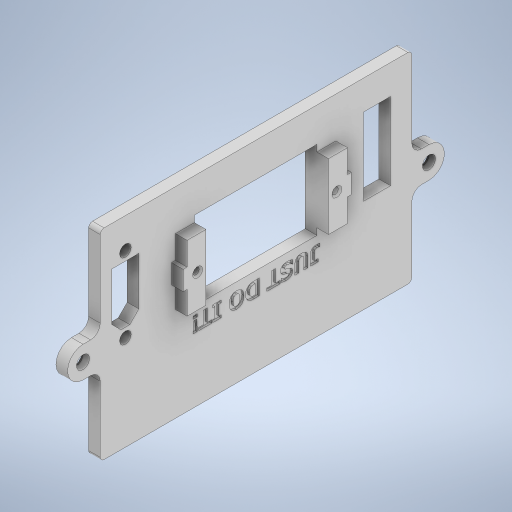
# Autodesk Inventor part: pokrywa_tyl
Saved by Autodesk Inventor 2023.4 (Build 274418000, 418)
## iProperties
Created: 2024-07-28
Part Number: pokrywa_tyl
Material: Ogólny
Document SubType Name: Modeling
Designer: kamil
Density: 1 g/cm^3
Appearance: Domyślna
Author: kamil
Autodesk Inventor part; units mm, degrees
ref_plane "YZ Plane" through (0, 0, 0) normal (1, 0, 0) x (0, 1, 0)
ref_plane "XZ Plane" through (0, 0, 0) normal (0, 1, 0) x (-1, 0, 0)
ref_plane "XY Plane" through (0, 0, 0) normal (0, 0, 1) x (1, 0, 0)
sketch "Szkic1" plane through (0, 0, 0) normal (1, 0, 0) x (0, 1, 0)
  line L0 (-29.4319, -23.6453) -> (19.8681, -23.6453)
  line L1 (19.8681, -23.6453) -> (19.8681, 56.9547)
  line L2 (19.8681, 56.9547) -> (-29.4319, 56.9547)
  line L3 (-29.4319, 56.9547) -> (-29.4319, -23.6453)
  point P0 (0, 0)
  dimension "d0" = 80.6
  dimension "d1" = 49.3
  constraints: 8 end point, 2 parallel, 1 horizontal, 1 perpendicular
  measures "d0" distance of L0.end L1.end
  measures "d1" distance between parallel lines of L3 L1
extrude "Wyciągnięcie proste1" add sketch "Szkic1" along normal blind 3
sketch "Sketch6" plane through (0, 0, 0) normal (-1, 0, 0) x (0, 0, 1)
  arc A0 (-28.0945, -0.5319) -> (-28.0945, -9.0319) centre (-28.0945, -4.7819) ccw
  line L0 (-26.3445, -9.0319) -> (-28.0945, -9.0319)
  line L1 (-26.3445, -0.5319) -> (-28.0945, -0.5319)
  line L2 (59.654, -6.3319) -> (61.404, -6.3319)
  arc A1 (61.404, -6.3319) -> (61.404, 2.1681) centre (61.404, -2.0819) ccw
  line L3 (59.654, 2.1681) -> (61.404, 2.1681)
  line L4 (-23.6453, 19.8681) -> (56.9547, 19.8681)
  line L5 (-23.6453, -29.4319) -> (-23.6453, 19.8681)
  line L6 (56.9547, -29.4319) -> (-23.6453, -29.4319)
  line L7 (56.9547, 19.8681) -> (56.9547, -29.4319)
  line L8 (-26.3445, -8.7819) -> (-28.0945, -8.7819)
  arc A2 (-28.0945, -0.7819) -> (-28.0945, -8.7819) centre (-28.0945, -4.7819) ccw
  line L9 (-28.0945, -0.7819) -> (-26.3445, -0.7819)
  line L10 (-26.3445, -0.7819) -> (-23.6453, -0.7819)
  line L11 (-23.6453, -29.4319) -> (-23.6453, 19.8681)
  line L12 (-26.3445, -8.7819) -> (-23.6453, -8.7819)
  line L13 (-23.6453, 19.8681) -> (56.9547, 19.8681)
  line L14 (16.6547, 19.8681) -> (16.6547, -29.4319)
  line L15 (56.9547, -29.4319) -> (-23.6453, -29.4319)
  line L16 (59.654, -8.7819) -> (61.404, -8.7819)
  arc A3 (61.404, -8.7819) -> (61.404, -0.7819) centre (61.404, -4.7819) ccw
  line L17 (61.404, -0.7819) -> (59.654, -0.7819)
  line L18 (59.654, -0.7819) -> (56.9547, -0.7819)
  line L19 (59.654, -8.7819) -> (56.9547, -8.7819)
  point P0 (0, 0)
extrude "Extrusion4" add sketch "Sketch6" against normal blind 3 contours L5 L12 L8 A2 L9 L10 | L18 L17 A3 L16 L19 L7
fillet "Fillet2" radius 2.5 4 edges at (1.5, -0.7819, -23.6453) (1.5, -8.7819, -23.6453) (1.5, -0.7819, 56.9547) (1.5, -8.7819, 56.9547)
sketch "Sketch8" plane through (0, 0, 0) normal (-1, 0, 0) x (0, 0, 1)
  line L0 (32.3929, 13.5523) -> (1.0929, 13.5523) projected
  line L1 (1.0929, 13.5523) -> (1.0929, -6.4477) projected
  line L2 (1.0929, -6.4477) -> (32.3929, -6.4477) projected
  line L3 (32.3929, -6.4477) -> (32.3929, 13.5523) projected
  line L4 (0.8929, -6.6477) -> (0.8929, 13.7523)
  line L5 (0.8929, 13.7523) -> (32.5929, 13.7523)
  line L6 (32.5929, 13.7523) -> (32.5929, -6.6477)
  line L7 (32.5929, -6.6477) -> (0.8929, -6.6477)
  point P0 (0, 0)
  dimension "d38" = 0.2
  constraints: 8 end point, 3 other
  measures "d38" distance between parallel lines of L1 L4
extrude "Extrusion5" cut sketch "Sketch8" against normal blind 3 contours L3 L2 L1 L0 | L4 L5 L6 L7
sketch "Sketch9" plane through (3, 0, 0) normal (1, 0, 0) x (0, 0, -1)
  line L0 (-32.5929, 13.7523) -> (-0.8929, 13.7523) projected
  line L1 (-0.8929, 13.7523) -> (-0.8929, -6.6477) projected
  line L2 (-0.8929, -6.6477) -> (-32.5929, -6.6477) projected
  line L3 (-32.5929, -6.6477) -> (-32.5929, 13.7523) projected
  line L4 (-56.9547, -29.4319) -> (23.6453, -29.4319) projected
  line L5 (23.6453, -29.4319) -> (23.6453, -11.2819) projected
  arc A0 (26.1453, -8.7819) -> (23.6453, -11.2819) centre (26.1453, -11.2819) ccw projected
  line L6 (26.1453, -8.7819) -> (28.0945, -8.7819) projected
  arc A1 (28.0945, -8.7819) -> (28.0945, -0.7819) centre (28.0945, -4.7819) ccw projected
  line L7 (28.0945, -0.7819) -> (26.1453, -0.7819) projected
  arc A2 (23.6453, 1.7181) -> (26.1453, -0.7819) centre (26.1453, 1.7181) ccw projected
  line L8 (23.6453, 1.7181) -> (23.6453, 19.8681) projected
  line L9 (23.6453, 19.8681) -> (-56.9547, 19.8681) projected
  line L10 (-56.9547, 19.8681) -> (-56.9547, 1.7181) projected
  line L11 (-37.4929, 12.0523) -> (-37.4929, 6.0523) projected
  line L12 (-37.4929, 6.0523) -> (-38.4929, 6.0523) projected
  line L13 (-38.4929, 6.0523) -> (-38.4929, 1.0523) projected
  line L14 (-38.4929, 1.0523) -> (-37.4929, 1.0523) projected
  line L15 (-37.4929, 1.0523) -> (-37.4929, -4.9477) projected
  line L16 (-37.4929, -4.9477) -> (4.0071, -4.9477) projected
  line L17 (4.0071, -4.9477) -> (4.0071, 1.0523) projected
  line L18 (4.0071, 1.0523) -> (5.0071, 1.0523) projected
  line L19 (5.0071, 1.0523) -> (5.0071, 6.0523) projected
  line L20 (5.0071, 6.0523) -> (4.0071, 6.0523) projected
  line L21 (4.0071, 6.0523) -> (4.0071, 12.0523) projected
  line L22 (4.0071, 12.0523) -> (-37.4929, 12.0523) projected
  circle A3 centre (1.2571, 3.5523) radius 1.2 projected
  circle A4 centre (-34.7429, 3.5523) radius 1.2 projected
  line L23 (-59.4547, -0.7819) -> (-61.404, -0.7819) projected
  arc A5 (-61.404, -0.7819) -> (-61.404, -8.7819) centre (-61.404, -4.7819) ccw projected
  line L24 (-61.404, -8.7819) -> (-59.4547, -8.7819) projected
  line L25 (-56.9547, -11.2819) -> (-56.9547, -29.4319) projected
  arc A6 (-59.4547, -0.7819) -> (-56.9547, 1.7181) centre (-59.4547, 1.7181) ccw projected
  arc A7 (-56.9547, -11.2819) -> (-59.4547, -8.7819) centre (-59.4547, -11.2819) ccw projected
  point P0 (0, 0)
  point P1 (-0.8929, 12.0523)
  point P2 (-0.8929, -4.9477)
  point P3 (-32.5929, -4.9477)
  point P4 (-32.5929, 12.0523)
ref_plane "Work Plane2" through (6, -4.9477, 32.3929) normal (-1, 0, 0) x (0, 0, 1)
extrude "Extrusion6" add sketch "Sketch9" along normal up to surface (3 mm away) contours L3 L16 L15 L14 L13 L12 L11 L22 | L22 L21 L20 L19 L18 L17 L16 L1 | A3 | A4
sketch "Sketch10" plane through (6, -4.9477, 32.5929) normal (1, 0, 0) x (0, 0, -1)
  circle A0 centre (33.85, 8.5) radius 1.2 projected
  circle A1 centre (-2.15, 8.5) radius 1.2 projected
  point P0 (32.5929, 4.9477)
hole "Hole4" at (6, 3.5523, -1.2571) at (6, 3.5523, 34.7429) direction (-1, 0, 0) diameter 1.7 depth 5 tip angle 118 countersink diameter 2.6 countersink angle 90
sketch "Sketch12" plane through (0, 0, 0) normal (-1, 0, 0) x (0, 0, 1)
  arc A0 (-28.0945, -0.7819) -> (-28.0945, -8.7819) centre (-28.0945, -4.7819) ccw projected
  arc A1 (61.404, -8.7819) -> (61.404, -0.7819) centre (61.404, -4.7819) ccw projected
  point P0 (0, 0)
hole "Hole5" at (0, -4.7819, -28.0945) at (0, -4.7819, 61.404) direction (1, 0, 0) diameter 3.4 depth 10 countersink diameter 6 countersink angle 90
sketch "Sketch13" plane through (0, -29.4319, -23.6453) normal (0, -1, 0) x (1, 0, 0)
  line L0 (0, 80.6) -> (0, 0) projected
  line L1 (0, 0) -> (3, 0) projected
  line L2 (3, 80.6) -> (3, 0) projected
  line L3 (0, 80.6) -> (3, 80.6) projected
  point P0 (0, 23.6453)
extrude "Extrusion8" add sketch "Sketch13" along normal blind 2.7
sketch "Sketch14" plane through (3, 0, 0) normal (1, 0, 0) x (0, 0, -1)
  line L0 (-56.9547, -11.2819) -> (-56.9547, -32.1319) projected
  line L1 (23.6453, -32.1319) -> (-56.9547, -32.1319) projected
  line L2 (23.6453, -11.2819) -> (23.6453, -32.1319) projected
  line L3 (-56.9547, -32.1319) -> (23.6453, -32.1319)
  line L4 (23.6453, -32.1319) -> (23.6453, -29.3319)
  line L5 (23.6453, -29.3319) -> (-56.9547, -29.3319)
  line L6 (-56.9547, -29.3319) -> (-56.9547, -32.1319)
  point P0 (0, 0)
  dimension "d70" = 2.8
  constraints: 8 end point, 2 parallel, 1 horizontal, 1 perpendicular, 1 point on line
  measures "d70" distance between parallel lines of L1 L5
extrude "Extrusion9" cut sketch "Sketch14" against normal through all
sketch "Sketch15" plane through (0, 19.8681, 56.9547) normal (0, 1, 0) x (1, 0, 0)
  line L0 (0, 80.6) -> (0, 0) projected
  line L1 (0, 0) -> (3, 0) projected
  line L2 (3, 80.6) -> (3, 0) projected
  line L3 (0, 80.6) -> (3, 80.6) projected
  point P0 (0, 56.9547)
extrude "Extrusion10" add sketch "Sketch15" along normal blind 2.7
fillet "Fillet7" radius 1 4 edges at (1.5, 22.5681, 56.9547) (1.5, 22.5681, -23.6453) (1.5, -29.3319, -23.6453) (1.5, -29.3319, 56.9547)
sketch "Sketch16" plane through (0, 0, 0) normal (-1, 0, 0) x (0, 0, 1)
  line L0 (-11.1453, -5.0319) -> (-18.1453, -5.0319)
  line L1 (-18.1453, -5.0319) -> (-18.1453, 14.9681)
  line L2 (-18.1453, 14.9681) -> (-11.1453, 14.9681)
  line L3 (-11.1453, 14.9681) -> (-11.1453, -5.0319)
  line L4 (50.4547, 14.7181) -> (50.4547, -4.7819) construction
  circle A0 centre (50.4547, 14.7181) radius 1.5
  circle A1 centre (50.4547, -4.7819) radius 1.5
  line L5 (53.9547, 12.3681) -> (53.9547, -2.4319)
  line L6 (53.9547, -2.4319) -> (46.9547, -2.4319)
  line L7 (46.9547, -2.4319) -> (46.9547, 12.3681)
  line L8 (46.9547, 12.3681) -> (53.9547, 12.3681)
  line L9 (50.4547, 8.5681) -> (50.4547, 1.3681)
  circle A2 centre (50.4547, 8.5681) radius 2.25
  circle A3 centre (50.4547, 1.3681) radius 2.25
  line L10 (46.9547, -0.0816) -> (49.305, -2.4319)
  line L11 (53.9547, -0.0816) -> (51.6045, -2.4319)
  circle A4 centre (50.4547, 1.3681) radius 3.5
  line L12 (56.9547, -11.2819) -> (56.9547, -28.3319) projected
  line L13 (-22.6453, -29.3319) -> (55.9547, -29.3319) projected
  line L14 (-23.6453, -11.2819) -> (-23.6453, -28.3319) projected
  circle A5 centre (61.404, -4.7819) radius 1.7 projected
  point P0 (0, 0)
  point P1 (50.4547, 4.9681)
  point P2 (53.9547, 4.9681)
  point P3 (50.4547, 4.9681)
  point P4 (50.4547, 12.3681)
  point P5 (13.6547, 4.9681)
  point P6 (-11.1453, 4.9681)
  point P7 (-14.6453, -5.0319)
  point P8 (16.6547, -29.3319)
  dimension "d76" = 7
  dimension "d77" = 20
  dimension "d78" = 19.5
  dimension "d79" = 3
  dimension "d80" = 3
  dimension "d81" = 14.8
  dimension "d82" = 7
  dimension "d83" = 7.2
  dimension "d84" = 4.5
  dimension "d85" = 4.5
  dimension "d86" = 45
  dimension "d87" = 45
  dimension "d98" = 3
  dimension "d99" = 45
  dimension "d101" = 5.5
  constraints: 24 end point, 7 midpoint, 5 centre point, 5 coincident, 5 horizontal alignment, 5 parallel, 4 point on line, 3 perpendicular, 3 tangent, 3 vertical alignment, 1 horizontal
  measures "d76" distance of L1.end L2.end
  measures "d77" distance of L0.end L1.end
  measures "d78" distance of L4.start L4.end
  measures "d79" diameter of A0
  measures "d80" diameter of A1
  measures "d81" distance of L6.end L7.end
  measures "d82" distance of L5.end L6.end
  measures "d83" distance of L9.start L9.end
  measures "d84" diameter of A2
  measures "d85" diameter of A3
  measures "d86" angle of L5 L11
  measures "d87" angle of L7 L10
  measures "d98" distance between parallel lines of L5 L12
  measures "d99" angle of L6 L11
  measures "d101" distance between parallel lines of L14 L1
extrude "Extrusion11" cut sketch "Sketch16" against normal through all contours L0 L1 L2 L3 | A0 | A1 | L5 A4 L7 L8 | A4 | L5 L11 A4 | L11 L6 L10 A4 | A4 L10 L7 | A2 | A3
sketch "Sketch17" plane through (3, 0, 0) normal (1, 0, 0) x (0, 0, -1)
  line L0 (5.0407, -18.26) -> (-38.5266, -18.26) construction
  line L1 (-38.5266, -18.26) -> (-38.5266, -3.1594) construction
  line L2 (-38.5266, -3.1594) -> (5.0407, -3.1594) construction
  line L3 (5.0407, -3.1594) -> (5.0407, -18.26) construction
  line L4 (-0.8929, -6.6477) -> (-32.5929, -6.6477) projected
  spline S0 degree 2 poles (-2.529, -9.8831) (-2.529, -9.6238) (-2.3507, -9.1635) (-2.1724, -9.0014) knots 0 0 0 1 2 2 2
  spline S1 degree 2 poles (-2.1724, -9.0014) (-1.9715, -8.8199) (-1.4237, -8.6481) (-1.0671, -8.6481) knots 0 0 0 1 2 2 2
  spline S2 degree 2 poles (-1.0671, -8.6481) (-0.8013, -8.6481) (-0.3345, -8.687) (-0.1562, -8.7259) knots 0 0 0 1 2 2 2
  line L5 (-0.1562, -8.7259) -> (-0.1562, -9.5362)
  line L6 (-0.1562, -9.5362) -> (-0.247, -9.5362)
  spline S3 degree 2 poles (-0.247, -9.5362) (-0.3669, -9.4876) (-0.6295, -9.4033) (-0.8369, -9.4033) knots 0 0 0 1 2 2 2
  spline S4 degree 2 poles (-0.8369, -9.4033) (-1.1028, -9.4033) (-1.3912, -9.5525) (-1.4496, -9.6886) knots 0 0 0 1 2 2 2
  spline S5 degree 2 poles (-1.4496, -9.6886) (-1.5112, -9.8215) (-1.5241, -10.1651) (-1.5241, -10.379) knots 0 0 0 1 2 2 2
  line L7 (-1.5241, -10.379) -> (-1.5241, -11.9836)
  line L8 (-1.5241, -11.9836) -> (-0.61, -11.9836)
  line L9 (-0.61, -11.9836) -> (-0.61, -12.7097)
  line L10 (-0.61, -12.7097) -> (-2.529, -12.7097)
  line L11 (-2.529, -12.7097) -> (-2.529, -9.8831)
  spline S6 degree 2 poles (-4.9245, -8.6254) (-4.1173, -8.6254) (-3.2486, -9.4033) (-3.2486, -10.1554) knots 0 0 0 1 2 2 2
  line L12 (-3.2486, -10.1554) -> (-3.2486, -12.7097)
  line L13 (-3.2486, -12.7097) -> (-4.2535, -12.7097)
  line L14 (-4.2535, -12.7097) -> (-4.2535, -10.2137)
  spline S7 degree 2 poles (-4.2535, -10.2137) (-4.2535, -9.7956) (-4.5679, -9.3871) (-4.9245, -9.3871) knots 0 0 0 1 2 2 2
  spline S8 degree 2 poles (-4.9245, -9.3871) (-5.2713, -9.3871) (-5.5955, -9.7794) (-5.5955, -10.2137) knots 0 0 0 1 2 2 2
  line L15 (-5.5955, -10.2137) -> (-5.5955, -12.7097)
  line L16 (-5.5955, -12.7097) -> (-6.6003, -12.7097)
  line L17 (-6.6003, -12.7097) -> (-6.6003, -10.1586)
  spline S9 degree 2 poles (-6.6003, -10.1586) (-6.6003, -9.4196) (-5.7543, -8.6254) (-4.9245, -8.6254) knots 0 0 0 1 2 2 2
  spline S10 degree 2 poles (-8.6068, -8.6384) (-8.1465, -8.6384) (-7.4528, -8.8166) (-7.1546, -8.9463) knots 0 0 0 1 2 2 2
  line L18 (-7.1546, -8.9463) -> (-7.1546, -9.8993)
  line L19 (-7.1546, -9.8993) -> (-7.2454, -9.8993)
  spline S11 degree 2 poles (-7.2454, -9.8993) (-7.5468, -9.6432) (-8.2697, -9.3677) (-8.61, -9.3677) knots 0 0 0 1 2 2 2
  spline S12 degree 2 poles (-8.61, -9.3677) (-8.6976, -9.3677) (-8.9796, -9.4066) (-9.0639, -9.4455) knots 0 0 0 1 2 2 2
  spline S13 degree 2 poles (-9.0639, -9.4455) (-9.1676, -9.4909) (-9.3134, -9.6562) (-9.3134, -9.7891) knots 0 0 0 1 2 2 2
  spline S14 degree 2 poles (-9.3134, -9.7891) (-9.3134, -9.9414) (-9.0768, -10.1294) (-8.9147, -10.1716) knots 0 0 0 1 2 2 2
  spline S15 degree 2 poles (-8.9147, -10.1716) (-8.7105, -10.2267) (-8.247, -10.3207) (-8.0428, -10.392) knots 0 0 0 1 2 2 2
  spline S16 degree 2 poles (-8.0428, -10.392) (-7.5792, -10.5541) (-7.1773, -11.1084) (-7.1773, -11.5233) knots 0 0 0 1 2 2 2
  spline S17 degree 2 poles (-7.1773, -11.5233) (-7.1773, -12.0841) (-8.1271, -12.781) (-8.8402, -12.781) knots 0 0 0 1 2 2 2
  spline S18 degree 2 poles (-8.8402, -12.781) (-9.1968, -12.781) (-9.9034, -12.6351) (-10.1822, -12.5119) knots 0 0 0 1 2 2 2
  line L20 (-10.1822, -12.5119) -> (-10.1822, -11.5978)
  line L21 (-10.1822, -11.5978) -> (-10.0946, -11.5978)
  spline S19 degree 2 poles (-10.0946, -11.5978) (-9.871, -11.7891) (-9.2292, -12.0516) (-8.8921, -12.0516) knots 0 0 0 1 2 2 2
  spline S20 degree 2 poles (-8.8921, -12.0516) (-8.7592, -12.0516) (-8.5517, -12.0127) (-8.435, -11.9609) knots 0 0 0 1 2 2 2
  spline S21 degree 2 poles (-8.435, -11.9609) (-8.341, -11.9187) (-8.2049, -11.7502) (-8.2049, -11.6465) knots 0 0 0 1 2 2 2
  spline S22 degree 2 poles (-8.2049, -11.6465) (-8.2049, -11.4909) (-8.422, -11.3126) (-8.7332, -11.2413) knots 0 0 0 1 2 2 2
  spline S23 degree 2 poles (-8.7332, -11.2413) (-8.9342, -11.1959) (-9.307, -11.1084) (-9.5209, -11.0338) knots 0 0 0 1 2 2 2
  spline S24 degree 2 poles (-9.5209, -11.0338) (-9.9358, -10.8815) (-10.341, -10.3758) (-10.341, -9.9609) knots 0 0 0 1 2 2 2
  spline S25 degree 2 poles (-10.341, -9.9609) (-10.341, -9.3644) (-9.4042, -8.6384) (-8.6068, -8.6384) knots 0 0 0 1 2 2 2
  line L22 (-11.6246, -8.7097) -> (-11.6246, -11.9479)
  line L23 (-11.6246, -11.9479) -> (-10.4415, -11.9479)
  line L24 (-10.4415, -11.9479) -> (-10.4415, -12.7097)
  line L25 (-10.4415, -12.7097) -> (-13.8126, -12.7097)
  line L26 (-13.8126, -12.7097) -> (-13.8126, -11.9479)
  line L27 (-13.8126, -11.9479) -> (-12.6295, -11.9479)
  line L28 (-12.6295, -11.9479) -> (-12.6295, -8.7097)
  line L29 (-12.6295, -8.7097) -> (-11.6246, -8.7097)
  spline S26 degree 2 poles (-19.4042, -10.7064) (-19.4042, -10.1456) (-18.9147, -9.264) (-18.542, -9.0273) knots 0 0 0 1 2 2 2
  spline S27 degree 2 poles (-18.542, -9.0273) (-18.2308, -8.8264) (-17.4982, -8.7097) (-17.0865, -8.7097) knots 0 0 0 1 2 2 2
  line L30 (-17.0865, -8.7097) -> (-15.8353, -8.7097)
  line L31 (-15.8353, -8.7097) -> (-15.8353, -12.7097)
  line L32 (-15.8353, -12.7097) -> (-17.0736, -12.7097)
  spline S28 degree 2 poles (-17.0736, -12.7097) (-17.495, -12.7097) (-18.2308, -12.6027) (-18.5549, -12.3952) knots 0 0 0 1 2 2 2
  spline S29 degree 2 poles (-18.5549, -12.3952) (-18.9472, -12.1424) (-19.4042, -11.2867) (-19.4042, -10.7064) knots 0 0 0 1 2 2 2
  spline S30 degree 2 poles (-18.3734, -10.7129) (-18.3734, -11.1084) (-18.1011, -11.6724) (-17.8224, -11.8312) knots 0 0 0 1 2 2 2
  spline S31 degree 2 poles (-17.8224, -11.8312) (-17.6181, -11.9414) (-17.1708, -11.9641) (-16.8596, -11.9641) knots 0 0 0 1 2 2 2
  line L33 (-16.8596, -11.9641) -> (-16.8402, -11.9641)
  line L34 (-16.8402, -11.9641) -> (-16.8402, -9.4584)
  line L35 (-16.8402, -9.4584) -> (-16.8596, -9.4584)
  spline S32 degree 2 poles (-16.8596, -9.4584) (-17.1968, -9.4584) (-17.6603, -9.4811) (-17.871, -9.614) knots 0 0 0 1 2 2 2
  spline S33 degree 2 poles (-17.871, -9.614) (-18.1173, -9.7696) (-18.3734, -10.3174) (-18.3734, -10.7129) knots 0 0 0 1 2 2 2
  spline S34 degree 2 poles (-23.6408, -10.7097) (-23.6408, -9.7372) (-22.6036, -8.6254) (-21.7024, -8.6254) knots 0 0 0 1 2 2 2
  spline S35 degree 2 poles (-21.7024, -8.6254) (-20.7981, -8.6254) (-19.7673, -9.7502) (-19.7673, -10.7097) knots 0 0 0 1 2 2 2
  spline S36 degree 2 poles (-19.7673, -10.7097) (-19.7673, -11.6724) (-20.7981, -12.7939) (-21.7024, -12.7939) knots 0 0 0 1 2 2 2
  spline S37 degree 2 poles (-21.7024, -12.7939) (-22.6036, -12.7939) (-23.6408, -11.6789) (-23.6408, -10.7097) knots 0 0 0 1 2 2 2
  spline S38 degree 2 poles (-22.6036, -10.7097) (-22.6036, -11.0695) (-22.4577, -11.5719) (-22.3313, -11.7307) knots 0 0 0 1 2 2 2
  spline S39 degree 2 poles (-22.3313, -11.7307) (-22.2049, -11.8961) (-21.8807, -12.0387) (-21.7057, -12.0387) knots 0 0 0 1 2 2 2
  spline S40 degree 2 poles (-21.7057, -12.0387) (-21.5209, -12.0387) (-21.2194, -11.9058) (-21.0801, -11.7372) knots 0 0 0 1 2 2 2
  spline S41 degree 2 poles (-21.0801, -11.7372) (-20.9569, -11.5816) (-20.8045, -11.0662) (-20.8045, -10.7097) knots 0 0 0 1 2 2 2
  spline S42 degree 2 poles (-20.8045, -10.7097) (-20.8045, -10.3401) (-20.9504, -9.8539) (-21.0768, -9.6886) knots 0 0 0 1 2 2 2
  spline S43 degree 2 poles (-21.0768, -9.6886) (-21.2032, -9.5233) (-21.5306, -9.3807) (-21.7057, -9.3807) knots 0 0 0 1 2 2 2
  spline S44 degree 2 poles (-21.7057, -9.3807) (-21.884, -9.3807) (-22.2146, -9.533) (-22.3345, -9.6951) knots 0 0 0 1 2 2 2
  spline S45 degree 2 poles (-22.3345, -9.6951) (-22.4642, -9.8701) (-22.6036, -10.3337) (-22.6036, -10.7097) knots 0 0 0 1 2 2 2
  line L36 (-27.8386, -8.7097) -> (-25.6862, -8.7097)
  line L37 (-25.6862, -8.7097) -> (-25.6862, -9.4066)
  line L38 (-25.6862, -9.4066) -> (-26.26, -9.4066)
  line L39 (-26.26, -9.4066) -> (-26.26, -12.0127)
  line L40 (-26.26, -12.0127) -> (-25.6862, -12.0127)
  line L41 (-25.6862, -12.0127) -> (-25.6862, -12.7097)
  line L42 (-25.6862, -12.7097) -> (-27.8386, -12.7097)
  line L43 (-27.8386, -12.7097) -> (-27.8386, -12.0127)
  line L44 (-27.8386, -12.0127) -> (-27.2648, -12.0127)
  line L45 (-27.2648, -12.0127) -> (-27.2648, -9.4066)
  line L46 (-27.2648, -9.4066) -> (-27.8386, -9.4066)
  line L47 (-27.8386, -9.4066) -> (-27.8386, -8.7097)
  line L48 (-29.2746, -8.7097) -> (-29.2746, -11.9479)
  line L49 (-29.2746, -11.9479) -> (-28.0914, -11.9479)
  line L50 (-28.0914, -11.9479) -> (-28.0914, -12.7097)
  line L51 (-28.0914, -12.7097) -> (-31.4626, -12.7097)
  line L52 (-31.4626, -12.7097) -> (-31.4626, -11.9479)
  line L53 (-31.4626, -11.9479) -> (-30.2794, -11.9479)
  line L54 (-30.2794, -11.9479) -> (-30.2794, -8.7097)
  line L55 (-30.2794, -8.7097) -> (-29.2746, -8.7097)
  line L56 (-32.9374, -12.7097) -> (-32.8272, -9.8636)
  line L57 (-32.8272, -9.8636) -> (-31.978, -9.8636)
  line L58 (-31.978, -9.8636) -> (-31.8677, -12.7097)
  line L59 (-31.8677, -12.7097) -> (-32.9374, -12.7097)
  line L60 (-32.931, -8.7097) -> (-31.8742, -8.7097)
  line L61 (-31.8742, -8.7097) -> (-31.8742, -9.4196)
  line L62 (-31.8742, -9.4196) -> (-32.931, -9.4196)
  line L63 (-32.931, -9.4196) -> (-32.931, -8.7097)
  point P0 (0, 0)
  point P1 (-16.7429, -6.6477)
  point P2 (-16.7429, -18.26)
  constraints: 2 midpoint, 1 vertical alignment, 2 other
extrude "Extrusion12" cut sketch "Sketch17" against normal blind 0.5
